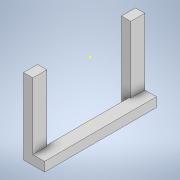
# Autodesk Inventor part: roof4
Saved by Autodesk Inventor 2020 (Build 240168000, 168)
## iProperties
Created: 2019-08-01
Part Number: roof4
Material: Generic
Document SubType Name: Modeling
Designer: cui_t
Density: 1 g/cm^3
Appearance: Default
Author: cui_t
Autodesk Inventor part; units mm, degrees
ref_plane "YZ Plane" through (0, 0, 0) normal (1, 0, 0) x (0, 1, 0)
ref_plane "XZ Plane" through (0, 0, 0) normal (0, 1, 0) x (-1, 0, 0)
ref_plane "XY Plane" through (0, 0, 0) normal (0, 0, 1) x (1, 0, 0)
sketch "Sketch1" plane through (0, 0, 0) normal (0, 1, 0) x (-1, 0, 0)
  line L0 (-4.5, 24) -> (4.5, 24)
  line L1 (4.5, 24) -> (4.5, -24)
  line L2 (4.5, -24) -> (-4.5, -24)
  line L3 (-4.5, -24) -> (-4.5, 24)
  line L4 (-4.5, 24) -> (4.5, -24) construction
  line L5 (4.5, 24) -> (-4.5, -24) construction
  point P0 (0, 0)
  dimension "d0" = 9
  dimension "d1" = 48
  constraints: 12 end point, 2 midpoint, 2 parallel, 1 horizontal, 1 perpendicular
  measures "d0" distance of L1.end L2.end
  measures "d1" distance of L0.end L1.end
extrude "Extrusion1" add sketch "Sketch1" along normal blind 4
sketch "Sketch2" plane through (0, 4, 0) normal (0, 1, 0) x (1, 0, 0)
  line L0 (4.5, 24) -> (-4.5, 24) projected
  line L1 (-4.5, 24) -> (-0.5, 24)
  line L2 (-0.5, 24) -> (-0.5, 18)
  line L3 (-0.5, 18) -> (-4.5, 18)
  line L4 (-4.5, 18) -> (-4.5, 24)
  line L5 (-4.5, -24) -> (4.5, -24) projected
  line L6 (-4.5, -24) -> (-0.5, -24)
  line L7 (-0.5, -24) -> (-0.5, -18)
  line L8 (-0.5, -18) -> (-4.5, -18)
  line L9 (-4.5, -18) -> (-4.5, -24)
  point P0 (0, 0)
  dimension "d4" = 4
  dimension "d5" = 6
  dimension "d6" = 4
  dimension "d7" = 6
  constraints: 16 end point, 4 parallel, 2 horizontal, 2 perpendicular
  measures "d4" distance of L2.end L3.end
  measures "d5" distance of L1.end L2.end
  measures "d6" distance of L8.end L7.end
  measures "d7" distance of L7.end L6.end
extrude "Extrusion2" add sketch "Sketch2" along normal blind 24.5
sketch "Sketch3" plane through (0, 4, 0) normal (0, 1, 0) x (1, 0, 0)
  point P0 (0, 0)
sketch "Sketch4" plane through (0, 4, 0) normal (0, 1, 0) x (1, 0, 0)
  line L0 (-4.5, 18) -> (1, 18)
  line L1 (1, 18) -> (1, -18)
  line L2 (1, -18) -> (-4.5, -18)
  line L3 (-4.5, -18) -> (-4.5, 18)
  line L4 (-4.5, 18) -> (-4.5, -18) projected
  line L5 (-4.5, -18) -> (-0.5, -18) projected
  point P0 (0, 0)
  dimension "d10" = 5.5
  dimension "d11" = 36
  constraints: 8 end point, 2 collinear, 2 parallel, 1 horizontal, 1 perpendicular
  measures "d10" distance of L1.end L2.end
  measures "d11" distance of L0.end L1.end
extrude "Extrusion3" cut sketch "Sketch4" against normal blind 4
sketch "Sketch5" plane through (1, 4, -18) normal (-1, 0, 0) x (0, 0, 1)
  line L0 (36, -4) -> (0, -4)
  line L1 (0, -4) -> (0, 0)
  line L2 (0, 0) -> (36, 0)
  line L3 (36, 0) -> (36, -4)
  line L4 (0, 0) -> (36, 0) projected
  line L5 (0, 0) -> (0, -4) projected
  point P0 (18, -4)
  dimension "d14" = 36
  dimension "d15" = 4
  constraints: 8 end point, 2 collinear, 2 parallel, 1 horizontal, 1 perpendicular
  measures "d14" distance of L1.end L2.end
  measures "d15" distance of L0.end L1.end
extrude "Extrusion4" add sketch "Sketch5" along normal blind 2
sketch "Sketch6" plane through (0, 28.5, 0) normal (0, 1, 0) x (1, 0, 0)
  point P0 (0, 0)
sketch "Sketch7" plane through (0, 28.5, 0) normal (0, 1, 0) x (1, 0, 0)
  line L0 (-4.5, -18) -> (-4.5, -24) projected
  line L1 (-0.5, -18) -> (-0.5, -24) projected
  line L2 (-4.5, -24) -> (-0.5, -24)
  line L3 (-0.5, -24) -> (-0.5, -18)
  line L4 (-0.5, -18) -> (-4.5, -18)
  line L5 (-4.5, -18) -> (-4.5, -24)
  line L6 (-4.5, 24) -> (-4.5, 18) projected
  line L7 (-0.5, 24) -> (-0.5, 18) projected
  line L8 (-4.5, 18) -> (-0.5, 18)
  line L9 (-0.5, 18) -> (-0.5, 24)
  line L10 (-0.5, 24) -> (-4.5, 24)
  line L11 (-4.5, 24) -> (-4.5, 18)
  point P0 (0, 0)
  constraints: 16 end point, 4 parallel, 2 horizontal, 2 perpendicular
extrude "Extrusion5" add sketch "Sketch7" along normal blind 4
body "Solid1"
